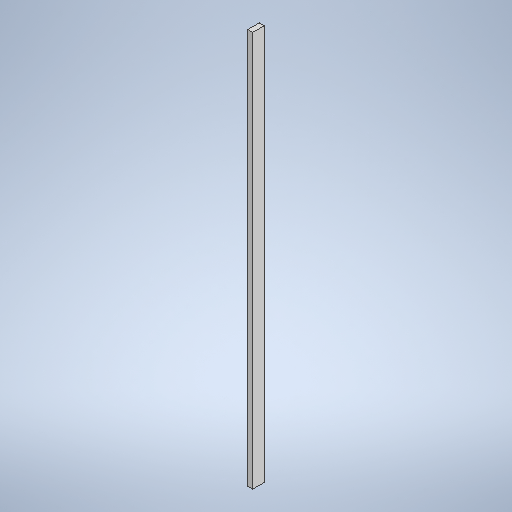
# Autodesk Inventor part: 10'x2x4
Saved by Autodesk Inventor 2025 (Build 290162000, 162)
## iProperties
Created: 2024-09-18
Part Number: 10'x2x4
Material: Generic
Document SubType Name: Modeling
Designer: localadmin
Density: 1 g/cm^3
Appearance: Default
Author: localadmin
Autodesk Inventor part; units mm, degrees
ref_plane "YZ Plane" through (0, 0, 0) normal (1, 0, 0) x (0, 1, 0)
ref_plane "XZ Plane" through (0, 0, 0) normal (0, 1, 0) x (-1, 0, 0)
ref_plane "XY Plane" through (0, 0, 0) normal (0, 0, 1) x (1, 0, 0)
sketch "Sketch1" plane through (0, 0, 0) normal (1, 0, 0) x (0, 1, 0)
  line L0 (0, 0) -> (3048, 0)
  line L1 (3048, 0) -> (3048, -88.9)
  line L2 (3048, -88.9) -> (0, -88.9)
  line L3 (0, -88.9) -> (0, 0)
  dimension "d0" = 3048
  dimension "d1" = 88.9
  constraints: 8 end point, 2 parallel, 1 horizontal, 1 perpendicular
  measures "d0" distance of L1.end L2.end
  measures "d1" distance of L0.end L1.end
extrude "Extrusion1" add sketch "Sketch1" along normal blind 38.1
body "Solid1"
